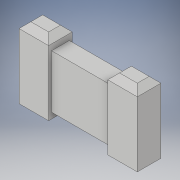
# Autodesk Inventor part: Wall
Saved by Autodesk Inventor 2019 (Build 230136000, 136)
## iProperties
Created: 2021-01-15
Part Number: Wall
Material: Generic
Document SubType Name: Modeling
Designer: Lee Gillan
Density: 1 g/cm^3
Appearance: Default
Author: Lee Gillan
Autodesk Inventor part; units mm, degrees
ref_plane "YZ Plane" through (0, 0, 0) normal (1, 0, 0) x (0, 1, 0)
sketch "Sketch1" plane through (0, 0, 0) normal (0, 1, 0) x (-1, 0, 0)
  line L0 (0, 0) -> (-2, 0)
  line L1 (-2, 0) -> (-2, -0.3)
  line L2 (-2, -0.3) -> (0, -0.3)
  line L3 (0, -0.3) -> (0, 0)
  dimension "d0" = 2
  dimension "d3" = 0.3
  constraints: 8 end point, 2 parallel, 1 horizontal, 1 perpendicular
  measures "d0" distance of L2.end L1.end
  measures "d3" distance of L0.end L1.end
extrude "Extrusion1" add sketch "Sketch1" along normal blind 1
ref_plane "Work Plane1" through (0, 0.5, 0) normal (0, 1, 0) x (1, 0, 0)
sketch "Sketch3" plane through (0, 0.5, 0) normal (0, 1, 0) x (1, 0, 0)
  line L0 (2, 0.3) -> (0, 0.3) projected
  line L1 (0, 0) -> (2, 0) projected
  line L2 (0, 0.3) -> (0.5, 0.3)
  line L3 (0.5, 0.3) -> (0.5, 0)
  line L4 (0.5, 0) -> (0, 0)
  line L5 (0, 0) -> (0, 0.3)
  line L6 (2, 0) -> (2, 0.3) projected
  line L7 (2, 0.3) -> (1.5, 0.3)
  line L8 (1.5, 0.3) -> (1.5, 0)
  line L9 (1.5, 0) -> (2, 0)
  line L10 (2, 0) -> (2, 0.3)
  dimension "d7" = 0.5
  dimension "d8" = 0.5
  constraints: 16 end point, 4 parallel, 2 horizontal, 2 perpendicular, 2 point on line
  measures "d7" distance of L3.end L4.end
  measures "d8" distance of L9.end L8.end
extrude "Extrusion2" add sketch "Sketch3" along normal mid plane 1.2 contours L6 L1 L8 L0 | L3 L1 L5 L0
ref_plane "Work Plane2" through (0.5, 0, -0.15) normal (0, 0, 1) x (1, 0, 0)
sketch "Sketch4" plane through (0.5, 0, -0.15) normal (0, 0, 1) x (1, 0, 0)
  line L0 (-0.5, -0.1) -> (-0.5, 1.1) projected
  line L1 (0, -0.1) -> (0, 0) projected
  line L2 (-0.5, 1.1) -> (0, 1.1)
  line L3 (0, 1.1) -> (0, -0.1)
  line L4 (0, -0.1) -> (-0.5, -0.1)
  line L5 (-0.5, -0.1) -> (-0.5, 1.1)
  line L6 (1.5, -0.1) -> (1, -0.1) projected
  line L7 (1.5, -0.1) -> (1.5, 1.1) projected
  line L8 (1, -0.1) -> (1.5, -0.1)
  line L9 (1.5, -0.1) -> (1.5, 1.1)
  line L10 (1.5, 1.1) -> (1, 1.1)
  line L11 (1, 1.1) -> (1, -0.1)
  point P0 (-0.5, 0)
  constraints: 16 end point, 4 parallel, 2 horizontal, 2 perpendicular
extrude "Extrusion3" add sketch "Sketch4" along normal mid plane 0.4
chamfer "Chamfer1" distance 0.1 angle 45 4 edges at (0.25, 1.1, 0.05) (0.25, 1.1, -0.35) (1.75, 1.1, 0.05) (1.75, 1.1, -0.35)
chamfer "Chamfer2" distance 0.1 angle 45 2 edges at (0, 1.1, -0.15) (2, 1.1, -0.15)
chamfer "Chamfer3" distance 0.1 angle 45 2 edges at (0.5, 1.1, -0.15) (1.5, 1.1, -0.15)
sketch "Sketch5" plane through (0, 1, 0) normal (0, 1, 0) x (1, 0, 0)
  line L0 (0.5, -0.05) -> (0.5, 0) projected
  line L1 (1.5, 0.3) -> (0.5, 0.3) projected
  line L2 (0.5, 0) -> (1.5, 0)
  line L3 (1.5, 0) -> (1.5, 0.3)
  line L4 (1.5, 0.3) -> (0.5, 0.3)
  line L5 (0.5, 0.3) -> (0.5, 0)
  point P0 (0, 0)
  constraints: 8 end point, 2 parallel, 1 horizontal, 1 perpendicular
extrude "Extrusion4" cut sketch "Sketch5" against normal blind 0.1
body "Solid1"
